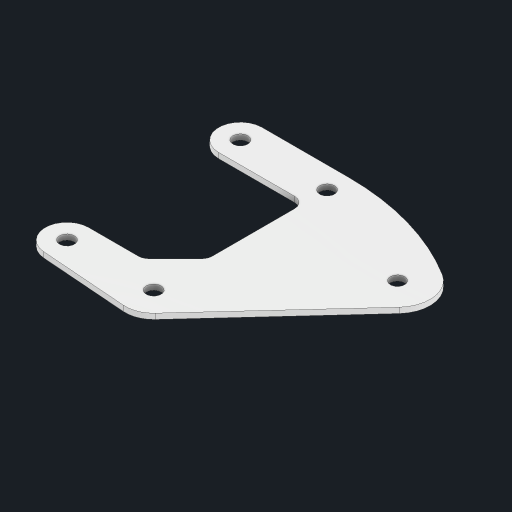
# Autodesk Inventor part: gusset
Saved by Autodesk Inventor 2024 (Build 280153000, 153)
## iProperties
Created: 2024-05-14
Part Number: gusset
Material: Acetal Resin, White
Document SubType Name: Modeling
Designer: Averey Ku
Density: 1.425 g/cm^3
Appearance: Smooth - White
d0: 0.375 in
d1: 0.375 in
d2: 0.125 in
d3: 0.165 in
d4: 0.125 in
Author: Averey Ku
Autodesk Inventor part; units mm, degrees
ref_plane "YZ Plane" through (0, 0, 0) normal (1, 0, 0) x (0, 1, 0)
ref_plane "XZ Plane" through (0, 0, 0) normal (0, 1, 0) x (-1, 0, 0)
ref_plane "XY Plane" through (0, 0, 0) normal (0, 0, 1) x (1, 0, 0)
sketch "main" plane through (0, 0, 0) normal (0, 0, 1) x (1, 0, 0)
  circle A0 centre (7.297, 24.2073) radius 2.1844
  arc A1 (32.7001, 17.8573) -> (32.7001, 30.5808) centre (32.7001, 24.219) ccw
  line L0 (8.227, 9.2622) -> (15.8921, 16.9273)
  arc A2 (18.1371, 17.8573) -> (15.8921, 16.9273) centre (18.1371, 14.6823) ccw
  line L1 (32.7001, 17.8573) -> (18.1371, 17.8573)
  circle A3 centre (32.697, 24.2073) radius 2.1844
  line L2 (7.9237, 32.4766) -> (33.1809, 30.5626)
  arc A4 (7.9237, 32.4766) -> (1.1906, 29.8185) centre (7.297, 24.2073) ccw
  circle A5 centre (7.297, -26.5927) radius 2.1844
  arc A6 (-33.054, -7.4479) -> (-31.0726, -21.98) centre (-26.0405, -13.8927) ccw
  line L3 (1.381, 30.0257) -> (-33.054, -7.4479)
  arc A7 (-31.0726, -21.98) -> (7.297, -32.9427) centre (7.297, 39.6854) ccw
  line L4 (7.297, -32.9427) -> (32.697, -32.9427)
  arc A8 (32.697, -32.9427) -> (32.697, -20.2427) centre (32.697, -26.5927) ccw
  circle A9 centre (-26.0405, -13.8927) radius 2.0955
  line L5 (7.297, 7.0171) -> (7.297, -17.0677)
  arc A10 (7.297, -17.0677) -> (10.472, -20.2427) centre (10.472, -17.0677) ccw
  line L6 (10.472, -20.2427) -> (32.697, -20.2427)
  circle A11 centre (32.697, -26.5927) radius 2.1844
  arc A12 (8.227, 9.2622) -> (7.297, 7.0171) centre (10.472, 7.0171) ccw
  point P0 (10.5963, 4.2161)
  point P1 (16.822, 17.8573)
  point P2 (7.297, 8.3323)
  point P3 (1.963, 30.5573)
  point P4 (7.297, 17.8573)
  dimension "d0" = 9.525
  dimension "d1" = 9.525
  dimension "d2" = 3.175
  dimension "d3" = 4.191
  dimension "d4" = 3.175
  measures "d0" distance of point (7.297, 8.332) point (7.297, 17.857)
  measures "d1" distance of point (16.822, 17.857) point (7.297, 17.857)
  measures "d2" radius of A2
  measures "d3" diameter of A9
  measures "d4" radius of A10
sketch "Sketch1" plane through (0, 0, 0) normal (0, 1, 0) x (-1, 0, 0)
  circle A0 centre (-25.4, 50.8) radius 2.1844
  arc A1 (0.0031, 44.45) -> (0.0031, 57.1735) centre (0.0031, 50.8118) ccw
  line L0 (-24.4701, 35.8549) -> (-16.8049, 43.5201)
  arc A2 (-14.5599, 44.45) -> (-16.8049, 43.5201) centre (-14.5599, 41.275) ccw
  line L1 (0.0031, 44.45) -> (-14.5599, 44.45)
  circle A3 centre (0, 50.8) radius 2.1844
  line L2 (-24.7734, 59.0693) -> (0.4838, 57.1553)
  arc A4 (-24.7734, 59.0693) -> (-31.5064, 56.4112) centre (-25.4, 50.8) ccw
  circle A5 centre (-25.4, 0) radius 2.1844
  arc A6 (-65.751, 19.1448) -> (-63.7696, 4.6127) centre (-58.7375, 12.7) ccw
  line L3 (-31.316, 56.6184) -> (-65.751, 19.1448)
  arc A7 (-63.7696, 4.6127) -> (-25.4, -6.35) centre (-25.4, 66.2781) ccw
  line L4 (-25.4, -6.35) -> (0, -6.35)
  arc A8 (0, -6.35) -> (0, 6.35) centre (0, 0) ccw
  circle A9 centre (-58.7375, 12.7) radius 2.0955
  line L5 (-25.4, 33.6099) -> (-25.4, 9.525)
  arc A10 (-25.4, 9.525) -> (-22.225, 6.35) centre (-22.225, 9.525) ccw
  line L6 (-22.225, 6.35) -> (0, 6.35)
  circle A11 centre (0, 0) radius 2.1844
  arc A12 (-24.4701, 35.8549) -> (-25.4, 33.6099) centre (-22.225, 33.6099) ccw
  constraints: 1 other
extrude "Extrusion1" add sketch "Sketch1" along normal blind 1.5875
equation "\"d1\" = d0"
body "Solid1"
